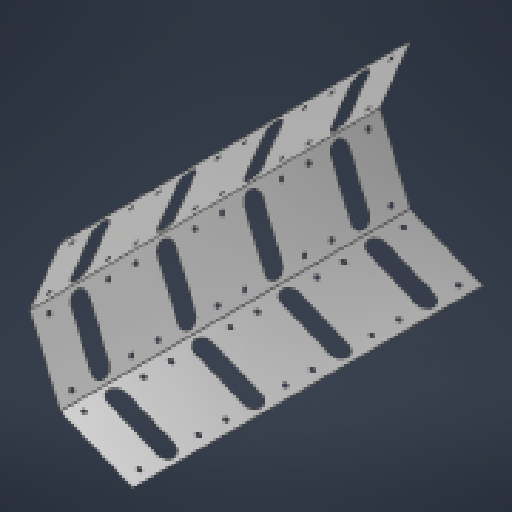
# Autodesk Inventor part: DMF 01 13 Барабан Лист лев брт v2.1
Saved by Autodesk Inventor 2026.2 (Build 302298010, 298A)
## iProperties
Created: 2024-04-28
Part Number: DMF 01 13 Барабан Лист лев брт v2.1
Material: Stainless Steel AISI 304
Document SubType Name: Sheet Metal
Designer: pokla
Density: 8 g/cm^3
Appearance: Chrome - Satin
Sheet Metal Rule: Default
Flat Pattern Width: 65.4696 cm
Flat Pattern Length: 97 cm
Flat Pattern Area: 6350.55 cm^2
Sheet Metal Width: 654,696 mm
Sheet Metal Length: 970,000 mm
Sheet Metal Area: 635055,159 mm^2
Stock Number: Барабан_Лист_Левый_Борт
d218: 145,000 mm
d219: 50,000 mm
d228: 145,000 mm
d229: 50,000 mm
Author: pokla
Autodesk Inventor part; units mm, degrees
ref_plane "YZ Plane" through (0, 0, 0) normal (1, 0, 0) x (0, 1, 0)
ref_plane "XZ Plane" through (0, 0, 0) normal (0, 1, 0) x (-1, 0, 0)
ref_plane "XY Plane" through (0, 0, 0) normal (0, 0, 1) x (1, 0, 0)
sketch "Sketch2" plane through (0, 0, 0) normal (0, 0, 1) x (1, 0, 0)
  line L0 (0, 286.8339) -> (202.8222, 202.8222) construction
  line L1 (202.8222, 202.8222) -> (286.8339, 0) construction
  line L2 (286.8339, 0) -> (202.8222, -202.8222) construction
  line L3 (202.8222, -202.8222) -> (0, -286.8339) construction
  line L4 (0, -286.8339) -> (-202.8222, -202.8222) construction
  line L5 (-202.8222, -202.8222) -> (-286.8339, 0) construction
  line L6 (-286.8339, 0) -> (-202.8222, 202.8222) construction
  line L7 (-202.8222, 202.8222) -> (0, 286.8339) construction
  line L8 (-286.1999, -1.5307) -> (-203.4563, -201.2915)
  line L9 (-201.2915, -203.4563) -> (-0.8315, -286.4895)
  arc A0 (-286.1999, 1.5307) -> (-286.1999, -1.5307) centre (-282.5044, 0) ccw
  arc A1 (-203.4563, -201.2915) -> (-201.2915, -203.4563) centre (-199.7608, -199.7608) ccw
  line L10 (-286.1999, 1.5307) -> (-203.1666, 201.9907)
  point P0 (0, 0)
  point P1 (0, 0)
  dimension "d58" = 4
  dimension "d59" = 4
  dimension "d70" = 0.9
  dimension "d72" = 0.9
  dimension "d74" = 530
  measures "d58" radius of A0
  measures "d59" radius of A1
  measures "d70" distance of L3.end L9.end
  measures "d72" distance of L6.end L10.end
  measures "d74" distance between parallel lines of L1 L8
contour flange "Contour Flange3" sketch "Sketch2" thickness 2 bend radius 2 width 970 along (0, 0, -1) mid plane no both sides no wall seen from (-101.0615, -244.9729, 0) lies toward (0.3826834, 0.9238795, 0) curves L9 A1 L8 A0 L10
bend "Bend6"
corner "Corner6"
sketch "Sketch15" plane through (-286.1999, -1.5307, -970) normal (-0.9238795, -0.3826834, 0) x (0, 0, 1)
  line L0 (0, -216.2195) -> (0, 0) projected
  line L1 (970, -216.2195) -> (970, 0) projected
  line L2 (820, -35.6097) -> (870, -35.6097)
  line L3 (870, -35.6097) -> (870, -180.6097)
  line L4 (870, -180.6097) -> (820, -180.6097)
  line L5 (820, -180.6097) -> (820, -35.6097)
  line L6 (820, -35.6097) -> (870, -180.6097) construction
  line L7 (870, -35.6097) -> (820, -180.6097) construction
  arc A0 (870, -35.6097) -> (820, -35.6097) centre (845, -35.6097) ccw
  arc A1 (820, -180.6097) -> (870, -180.6097) centre (845, -180.6097) ccw
  circle A2 centre (762.5, -25.6097) radius 5.5
  circle A3 centre (927.5, -25.6097) radius 5.5
  line L8 (845, -35.6097) -> (845, -180.6097) construction
  line L9 (870, -108.1097) -> (820, -108.1097) construction
  circle A4 centre (762.5, -190.6097) radius 5.5
  circle A5 centre (927.5, -190.6097) radius 5.5
  circle A6 centre (762.5, -25.6097) radius 6.5
  circle A7 centre (845, -25.6097) radius 6.5
  circle A8 centre (845, -190.6097) radius 6.5
  circle A9 centre (762.5, -190.6097) radius 6.5
  circle A10 centre (927.5, -190.6097) radius 6.5
  circle A11 centre (927.5, -25.6097) radius 6.5
  point P0 (0, -108.1097)
  point P1 (845, -108.1097)
  point P2 (845, -108.1097)
  point P3 (970, -108.1097)
  dimension "d220" = 145
  dimension "d221" = 50
  dimension "d222" = 165
  dimension "d223" = 165
  dimension "d224" = 11
  dimension "d225" = 13
  dimension "d226" = 13
  dimension "d227" = 165
  dimension "d230" = 100
  constraints: 16 end point, 12 centre point, 7 midpoint, 4 coincident, 4 point on circle, 4 tangent, 3 equal radius, 2 parallel, 2 point on line, 1 horizontal, 1 horizontal alignment, 1 perpendicular, 1 vertical, 4 other
  measures "d220" distance of L2.end L3.end
  measures "d221" distance of L2.start L2.end
  measures "d222" distance of A3.centre A2.centre
  measures "d223" distance of A5.centre A3.centre
  measures "d224" diameter of A2
  measures "d225" diameter of A6
  measures "d226" diameter of A7
  measures "d227" distance of A8.centre A7.centre
  measures "d230" distance between parallel lines of L1 L3
extrude "Cut1" cut sketch "Sketch15" against normal through all contours A0 L2 | L2 L3 L4 L5 | L4 A1 | A2 | A3 | A4 | A5 | A6 | A7 | A8 | A9 | A10 | A11
pattern_linear "Rectangular Pattern3" count 4 spacing 240 along (0, 0, -1) of "Cut1"
pattern_circular "Circular Pattern3" count 3 over 90 about axis through (0, 0, -10) along (0, 0, 1) of "Cut1", "Rectangular Pattern3" both ways yes
equation "\"d58\" = BendRadius + Thickness"
equation "\"d59\" = BendRadius + Thickness"
equation "\"d74\" = Барабан_размер_по_плоскостям"
equation "\"d75\" = Thickness"
equation "\"d76\" = BendReliefWidth"
equation "\"d77\" = BendReliefDepth"
equation "\"d78\" = MinimumRemnant"
equation "\"d79\" = TransitionRadius"
equation "\"d81\" = BendRadius"
equation "\"d83\" = CornerReliefSize"
equation "\"d84\" = GapSize"
equation "\"d85\" = JacobiRadiusSize"
equation "\"BendRadius\" = Thickness"
equation "\"BendReliefWidth\" = Thickness"
equation "\"BendReliefDepth\" = 0.5 * Thickness"
equation "\"CornerReliefSize\" = 4 * Thickness"
equation "\"MinimumRemnant\" = 2 * Thickness"
equation "\"TransitionRadius\" = BendRadius"
equation "\"JacobiRadiusSize\" = BendRadius"
equation "\"GapSize\" = Thickness"
equation "\"Барабан_Середина_листа\" = 206.27835"
equation "\"d218\" = 145"
equation "\"d228\" = 145"
equation "\"Thickness\" = 2"
equation "\"Барабан_размер_по_плоскостям\" = 530"
body "Solid3"
